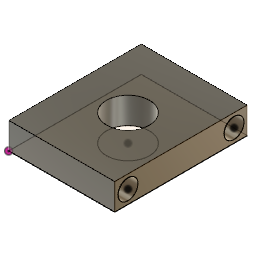
Hub Adapter (Autodesk Fusion 360 design; units mm, degrees)
Autodesk Fusion 360 part; units mm, degrees
sketch "Top" plane through (0, 0, 0) normal (0, 0, 1) x (1, 0, 0)
  line L0 (0, 0) -> (40, 0)
  line L1 (40, 0) -> (40, 50)
  line L2 (40, 50) -> (0, 50)
  line L3 (0, 50) -> (0, 0)
  circle A0 centre (20, 25) radius 8.1
  dimension "d6" = 40
  dimension "d7" = 50
  dimension "d11" = 16.2
  dimension "d12" = 25
  dimension "d13" = 20
  constraint horizontal L0
  constraint vertical L1
  constraint horizontal L2
  constraint vertical L3
  constraint coincident L0.start L3.end
  measures "d6" distance of L0.start L0.end
  measures "d7" distance of L0.start L2.end
  measures "d11" diameter of A0
  measures "d12" distance of L2 A0.centre
  measures "d13" distance of L1 A0.centre
extrude "Extrude1" add sketch "Top" along normal blind 10 contours L0 L1 L2 L3 | A0
extrude "Extrude2" cut sketch "Top" along normal blind 20 contours A0
sketch "Sketch2" plane through (40, 0, 0) normal (1, 0, 0) x (0, 1, 0)
  line L0 (0, 0) -> (50, 0)
  line L1 (50, 0) -> (50, 10)
  line L2 (50, 10) -> (0, 10)
  line L3 (0, 10) -> (0, 0)
  circle A0 centre (5, 5) radius 3.75
  circle A1 centre (45, 5) radius 3.75
  dimension "d16" = 7.5
  dimension "d17" = 7.5
  dimension "d18" = 5
  dimension "d19" = 5
  dimension "d20" = 5
  dimension "d21" = 5
  measures "d16" diameter of A0
  measures "d17" diameter of A1
  measures "d18" distance of L2 A0.centre
  measures "d19" distance of L3 A0.centre
  measures "d20" distance of L1 A1.centre
  measures "d21" distance of L2 A1.centre
extrude "Extrude3" cut sketch "Sketch2" against normal blind 50 contours A0
extrude "Extrude4" cut sketch "Sketch2" against normal blind 50 contours A1
equation "length = 50 mm"
equation "width = 40 mm"
equation "thickness = 10 mm"
equation "extra = 10 mm"
equation "fit_gap = 0.2 mm"
equation "d6 = width"
equation "d7 = length"
equation "d8 = thickness"
equation "bearing_8155_outer_radius = 8 mm"
equation "d11 = ( bearing_8155_outer_radius * 2 ) + fit_gap"
equation "d12 = length / 2"
equation "d13 = width / 2"
equation "d14 = thickness + extra"
equation "d16 = 3 * thickness / 4"
equation "d17 = 3 * thickness / 4"
equation "d18 = thickness / 2"
equation "d19 = thickness / 2"
equation "d20 = thickness / 2"
equation "d21 = thickness / 2"
equation "d22 = -( width + extra )"
equation "d24 = -( width + extra )"
